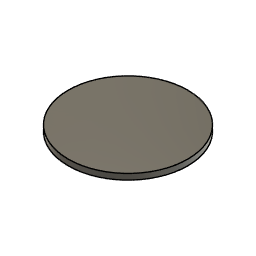
无标题 (Autodesk Fusion 360 design; units mm, degrees)
Autodesk Fusion 360 part; units mm, degrees
sketch "草图1" plane through (0, 0, 0) normal (0, 1, 0) x (1, 0, 0)
  circle A0 centre (0, 0) radius 51.5978
  constraint coincident A0.centre origin
extrude "拉伸1" add sketch "草图1" along normal blind 5
